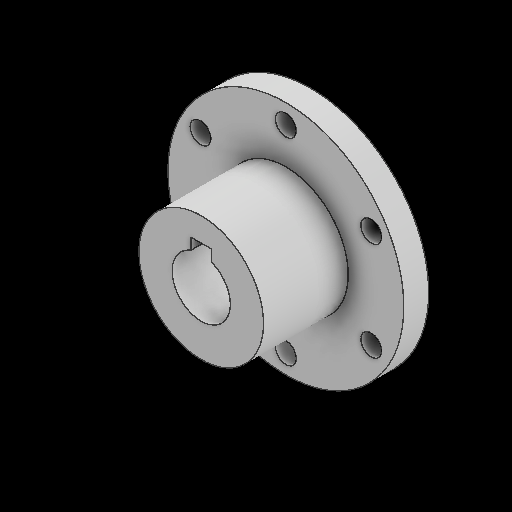
# Autodesk Inventor part: NexusRobot14mmKeywayHub
Saved by Autodesk Inventor 2025.2 (Build 292293000, 293)
## iProperties
Created: 2026-01-25
Part Number: NexusRobot14mmKeywayHub
Material: Generic
Document SubType Name: Modeling
Designer: LattePanda
Density: 1 g/cm^3
Appearance: Default
Author: LattePanda
Autodesk Inventor part; units mm, degrees
ref_plane "YZ Plane" through (0, 0, 0) normal (1, 0, 0) x (0, 1, 0)
ref_plane "XZ Plane" through (0, 0, 0) normal (0, 1, 0) x (-1, 0, 0)
ref_plane "XY Plane" through (0, 0, 0) normal (0, 0, 1) x (1, 0, 0)
sketch "Base" plane through (0, 0, 0) normal (0, 0, 1) x (1, 0, 0)
  circle A0 centre (0, 0) radius 28.4
  circle A1 centre (0, 0) radius 23.75 construction
  circle A2 centre (0, 0) radius 7
  line L0 (-2.5, 0) -> (2.5, 0)
  line L1 (2.5, 0) -> (2.5, 9.3)
  line L2 (2.5, 9.3) -> (-2.5, 9.3)
  line L3 (-2.5, 9.3) -> (-2.5, 0)
  line L4 (0, -39.76) -> (0, 39.76) construction
  circle A3 centre (0, 23.75) radius 2.5
  circle A4 centre (-20.5681, 11.875) radius 2.5
  circle A5 centre (-20.5681, -11.875) radius 2.5
  circle A6 centre (0, -23.75) radius 2.5
  circle A7 centre (20.5681, -11.875) radius 2.5
  circle A8 centre (20.5681, 11.875) radius 2.5
  point P0 (0, 9.3)
  point P1 (2.5, 6.5383)
  point P2 (-2.5, 6.5383)
  dimension "d1" = 47.5
  dimension "d0" = 56.8
  dimension "d2" = 14
  dimension "d3" = 9.3
  dimension "d4" = 5
  dimension "d5" = 5
  dimension "d8" = 360
  constraints: 8 centre point, 8 end point, 3 coincident, 2 midpoint, 2 parallel, 2 point on line, 1 horizontal, 1 perpendicular, 1 vertical alignment, 15 other
  measures "d0" diameter of A0
  measures "d2" diameter of A2
  measures "d3" distance of L0.end L1.end
  measures "d4" distance of L1.end L2.end
  measures "d5" diameter of A3
extrude "BaseFeature" add sketch "Base" along normal blind 6
sketch "Lip" plane through (0, 0, 6) normal (0, 0, 1) x (1, 0, 0)
  arc A0 (-2.5, 6.5383) -> (2.5, 6.5383) centre (0, 0) ccw projected
  circle A1 centre (0, 0) radius 15
  line L0 (-2.5, 6.5383) -> (-2.5, 9.3) projected
  line L1 (2.5, 9.3) -> (2.5, 6.5383) projected
  line L2 (-2.5, 9.3) -> (2.5, 9.3) projected
  dimension "d12" = 30
  constraints: 1 centre point, 1 coincident
  measures "d12" diameter of A1
extrude "LipFeature" add sketch "Lip" along normal blind 20.4
body "Solid1"
